Autodesk Inventor part; units mm, degrees
(part 2 of 2)
  line L952 (0.1814, -11.5919) -> (0.1714, -11.711)
  line L953 (0.1714, -11.711) -> (0.1647, -11.8346)
  line L954 (0.1647, -11.8346) -> (0.1634, -11.9625)
  line L955 (-2.9506, -10.7687) -> (-2.9407, -10.8745)
  line L956 (-2.9924, -10.5673) -> (-2.9697, -10.6658)
  line L957 (0.5555, -10.738) -> (0.49, -10.8119)
  line L958 (0.49, -10.8119) -> (0.4304, -10.8914)
  line L959 (0.4304, -10.8914) -> (0.3766, -10.9764)
  line L960 (0.3766, -10.9764) -> (0.331, -11.0665)
  line L961 (0.331, -11.0665) -> (0.2878, -11.1619)
  line L962 (0.2878, -11.1619) -> (0.2528, -11.2622)
  line L963 (1.245, -10.4259) -> (1.2243, -10.4284)
  line L964 (1.2656, -10.4234) -> (1.245, -10.4259)
  line L965 (1.2037, -10.4308) -> (1.183, -10.4331)
  line L966 (1.2243, -10.4284) -> (1.2037, -10.4308)
  line L967 (1.183, -10.4331) -> (1.1624, -10.4355)
  line L968 (0.6288, -10.67) -> (0.5555, -10.738)
  line L969 (0.7079, -10.6083) -> (0.6288, -10.67)
  line L970 (0.7968, -10.5532) -> (0.7079, -10.6083)
  line L971 (0.8944, -10.5055) -> (0.7968, -10.5532)
  line L972 (1.0105, -10.4657) -> (0.8944, -10.5055)
  line L973 (1.1624, -10.4355) -> (1.0105, -10.4657)
  line L974 (-3.7234, -9.8177) -> (-3.7039, -9.825)
  line L975 (-3.626, -9.8541) -> (-3.4858, -9.9197)
  line L976 (-3.4858, -9.9197) -> (-3.3825, -9.9862)
  line L977 (-3.3825, -9.9862) -> (-3.2992, -10.0559)
  line L978 (-3.2992, -10.0559) -> (-3.2261, -10.1307)
  line L979 (-3.2261, -10.1307) -> (-3.164, -10.2095)
  line L980 (-3.164, -10.2095) -> (-3.1091, -10.293)
  line L981 (-3.1091, -10.293) -> (-3.0632, -10.3804)
  line L982 (-3.0632, -10.3804) -> (-3.0244, -10.4719)
  line L983 (-3.0244, -10.4719) -> (-2.9924, -10.5673)
  line L984 (-2.9697, -10.6658) -> (-2.9506, -10.7687)
  line L985 (-3.6455, -9.8469) -> (-3.626, -9.8541)
  line L986 (-3.665, -9.8396) -> (-3.6455, -9.8469)
  line L987 (-3.7039, -9.825) -> (-3.6844, -9.8323)
  line L988 (-3.6844, -9.8323) -> (-3.665, -9.8396)
  line L989 (-2.9407, -10.8745) -> (-2.9384, -10.9833)
  line L990 (-2.7491, -14.0774) -> (-2.693, -14.2225)
  line L991 (-2.6334, -14.3678) -> (-2.5704, -14.5132)
  line L992 (-2.5704, -14.5132) -> (-2.504, -14.6587)
  line L993 (-2.504, -14.6587) -> (-2.3621, -14.6822)
  line L994 (-2.3621, -14.6822) -> (-2.22, -14.7044)
  line L995 (-2.22, -14.7044) -> (-2.0777, -14.7251)
  line L996 (-2.0777, -14.7251) -> (-1.9352, -14.7446)
  line L997 (-1.9352, -14.7446) -> (-1.7925, -14.7626)
  line L998 (-1.0768, -14.832) -> (-1.2202, -14.8209)
  line L999 (-1.2202, -14.8209) -> (-1.3635, -14.8084)
  line L1000 (-1.3635, -14.8084) -> (-1.5066, -14.7945)
  line L1001 (-1.5066, -14.7945) -> (-1.6496, -14.7792)
  line L1002 (-1.6496, -14.7792) -> (-1.7925, -14.7626)
  line L1003 (-2.8017, -13.9324) -> (-2.7491, -14.0774)
  line L1004 (3.5714, -13.2094) -> (3.6719, -13.3187)
  line L1005 (6.0773, -12.5539) -> (6.0676, -12.7049)
  line L1006 (6.0546, -12.8571) -> (6.0381, -13.0104)
  line L1007 (6.0381, -13.0104) -> (6.0184, -13.1648)
  line L1008 (6.0184, -13.1648) -> (5.9953, -13.3201)
  line L1009 (6.0676, -12.7049) -> (6.0546, -12.8571)
  line L1010 (5.9953, -13.3201) -> (5.9689, -13.4764)
  line L1011 (5.9689, -13.4764) -> (5.9393, -13.6335)
  line L1012 (6.0835, -12.4041) -> (6.0773, -12.5539)
  line L1013 (6.0862, -12.2556) -> (6.0835, -12.4041)
  line L1014 (6.0854, -12.1085) -> (6.0862, -12.2556)
  line L1015 (6, -11.2615) -> (6.0246, -11.3978)
  line L1016 (6.0246, -11.3978) -> (6.0447, -11.5363)
  line L1017 (6.0447, -11.5363) -> (6.0607, -11.6767)
  line L1018 (6.0607, -11.6767) -> (6.0727, -11.819)
  line L1019 (6.0727, -11.819) -> (6.0809, -11.963)
  line L1020 (6.0809, -11.963) -> (6.0854, -12.1085)
  line L1021 (2.6723, -11.5301) -> (2.7042, -11.654)
  line L1022 (2.7042, -11.654) -> (2.7296, -11.7839)
  line L1023 (2.7296, -11.7839) -> (2.7506, -11.9191)
  line L1024 (2.7506, -11.9191) -> (2.7948, -12.0443)
  line L1025 (2.7948, -12.0443) -> (2.8489, -12.1672)
  line L1026 (2.8489, -12.1672) -> (2.9098, -12.2884)
  line L1027 (2.9098, -12.2884) -> (2.9767, -12.4081)
  line L1028 (2.9767, -12.4081) -> (3.0487, -12.5264)
  line L1029 (3.0487, -12.5264) -> (3.1254, -12.6434)
  line L1030 (3.1254, -12.6434) -> (3.2066, -12.7592)
  line L1031 (3.2066, -12.7592) -> (3.2919, -12.8736)
  line L1032 (2.598, -11.2985) -> (2.6362, -11.4117)
  line L1033 (2.6362, -11.4117) -> (2.6723, -11.5301)
  line L1034 (2.5533, -11.1915) -> (2.598, -11.2985)
  line L1035 (5.704, -10.5164) -> (5.7711, -10.6304)
  line L1036 (5.7711, -10.6304) -> (5.845, -10.7456)
  line L1037 (5.845, -10.7456) -> (5.8949, -10.8686)
  line L1038 (5.8949, -10.8686) -> (5.9359, -10.9964)
  line L1039 (5.9359, -10.9964) -> (5.9707, -11.1276)
  line L1040 (5.9707, -11.1276) -> (6, -11.2615)
  line L1041 (3.2919, -12.8736) -> (3.3813, -12.9868)
  line L1042 (3.3813, -12.9868) -> (3.4745, -13.0987)
  line L1043 (3.4745, -13.0987) -> (3.5714, -13.2094)
  line L1044 (3.6719, -13.3187) -> (3.7758, -13.4267)
  line L1045 (3.7758, -13.4267) -> (3.8832, -13.5333)
  line L1046 (3.8832, -13.5333) -> (3.9939, -13.6386)
  line L1047 (4.225, -13.8449) -> (4.3453, -13.9459)
  line L1048 (2.5024, -11.0908) -> (2.5533, -11.1915)
  line L1049 (5.4577, -9.8547) -> (5.4815, -9.961)
  line L1050 (5.4815, -9.961) -> (5.5101, -10.0701)
  line L1051 (5.5101, -10.0701) -> (5.5476, -10.1798)
  line L1052 (5.5476, -10.1798) -> (5.5941, -10.2899)
  line L1053 (5.5941, -10.2899) -> (5.6456, -10.4025)
  line L1054 (5.6456, -10.4025) -> (5.704, -10.5164)
  line L1055 (2.3918, -10.9064) -> (2.4497, -10.9955)
  line L1056 (2.2612, -10.7475) -> (2.3271, -10.8242)
  line L1057 (5.4821, -9.2499) -> (5.4584, -9.3457)
  line L1058 (5.4584, -9.3457) -> (5.4426, -9.4438)
  line L1059 (5.4426, -9.4438) -> (5.4344, -9.5441)
  line L1060 (5.4344, -9.5441) -> (5.4359, -9.6451)
  line L1061 (5.4359, -9.6451) -> (5.442, -9.7497)
  line L1062 (5.442, -9.7497) -> (5.4577, -9.8547)
  line L1063 (5.9476, -8.6531) -> (5.9304, -8.6649)
  line L1064 (5.9647, -8.6413) -> (5.9476, -8.6531)
  line L1065 (5.9132, -8.6766) -> (5.896, -8.6883)
  line L1066 (5.9304, -8.6649) -> (5.9132, -8.6766)
  line L1067 (5.896, -8.6883) -> (5.8788, -8.7)
  line L1068 (5.5154, -9.1556) -> (5.4821, -9.2499)
  line L1069 (5.5568, -9.0642) -> (5.5154, -9.1556)
  line L1070 (5.6099, -8.9741) -> (5.5568, -9.0642)
  line L1071 (5.6741, -8.8865) -> (5.6099, -8.9741)
  line L1072 (5.7584, -8.7973) -> (5.6741, -8.8865)
  line L1073 (5.8788, -8.7) -> (5.7584, -8.7973)
  line L1074 (1.2656, -10.4234) -> (1.2863, -10.4209)
  line L1075 (1.3688, -10.4104) -> (1.5234, -10.4034)
  line L1076 (1.5234, -10.4034) -> (1.6458, -10.4143)
  line L1077 (1.6458, -10.4143) -> (1.7519, -10.4373)
  line L1078 (1.7519, -10.4373) -> (1.8514, -10.4695)
  line L1079 (1.8514, -10.4695) -> (1.943, -10.5104)
  line L1080 (1.943, -10.5104) -> (2.0304, -10.5589)
  line L1081 (2.0304, -10.5589) -> (2.1117, -10.615)
  line L1082 (2.1117, -10.615) -> (2.1885, -10.6779)
  line L1083 (2.1885, -10.6779) -> (2.2612, -10.7475)
  line L1084 (2.3271, -10.8242) -> (2.3918, -10.9064)
  line L1085 (1.3482, -10.4131) -> (1.3688, -10.4104)
  line L1086 (1.3275, -10.4157) -> (1.3482, -10.4131)
  line L1087 (1.2863, -10.4209) -> (1.3069, -10.4183)
  line L1088 (1.3069, -10.4183) -> (1.3275, -10.4157)
  line L1089 (2.4497, -10.9955) -> (2.5024, -11.0908)
  line L1090 (4.1079, -13.7425) -> (4.225, -13.8449)
  line L1091 (4.3453, -13.9459) -> (4.4687, -14.0453)
  line L1092 (4.4687, -14.0453) -> (4.595, -14.1433)
  line L1093 (4.595, -14.1433) -> (4.7316, -14.0982)
  line L1094 (4.7316, -14.0982) -> (4.8677, -14.0518)
  line L1095 (4.8677, -14.0518) -> (5.0034, -14.004)
  line L1096 (5.0034, -14.004) -> (5.1386, -13.955)
  line L1097 (5.1386, -13.955) -> (5.2733, -13.9046)
  line L1098 (5.9393, -13.6335) -> (5.8072, -13.6903)
  line L1099 (5.8072, -13.6903) -> (5.6745, -13.7458)
  line L1100 (5.6745, -13.7458) -> (5.5413, -13.8)
  line L1101 (5.5413, -13.8) -> (5.4076, -13.853)
  line L1102 (5.4076, -13.853) -> (5.2733, -13.9046)
  line L1103 (3.9939, -13.6386) -> (4.1079, -13.7425)
  line L1104 (9.301, -10.0366) -> (9.4408, -10.0867)
  line L1105 (11.2152, -8.2916) -> (11.2769, -8.4299)
  line L1106 (11.336, -8.5707) -> (11.3927, -8.7141)
  line L1107 (11.3927, -8.7141) -> (11.447, -8.8599)
  line L1108 (11.447, -8.8599) -> (11.4987, -9.0082)
  line L1109 (11.2769, -8.4299) -> (11.336, -8.5707)
  line L1110 (11.4987, -9.0082) -> (11.548, -9.1588)
  line L1111 (11.548, -9.1588) -> (11.5948, -9.3117)
  line L1112 (11.1511, -8.1561) -> (11.2152, -8.2916)
  line L1113 (11.0845, -8.0234) -> (11.1511, -8.1561)
  line L1114 (11.0155, -7.8936) -> (11.0845, -8.0234)
  line L1115 (10.5462, -7.1832) -> (10.6313, -7.2925)
  line L1116 (10.6313, -7.2925) -> (10.7135, -7.4057)
  line L1117 (10.7135, -7.4057) -> (10.793, -7.5227)
  line L1118 (10.793, -7.5227) -> (10.8697, -7.6431)
  line L1119 (10.8697, -7.6431) -> (10.9439, -7.7667)
  line L1120 (10.9439, -7.7667) -> (11.0155, -7.8936)
  line L1121 (7.7245, -8.9675) -> (7.8103, -9.0624)
  line L1122 (7.8103, -9.0624) -> (7.8932, -9.1656)
  line L1123 (7.8932, -9.1656) -> (7.9747, -9.2756)
  line L1124 (7.9747, -9.2756) -> (8.072, -9.3659)
  line L1125 (8.072, -9.3659) -> (8.1769, -9.4496)
  line L1126 (8.1769, -9.4496) -> (8.2872, -9.5285)
  line L1127 (8.2872, -9.5285) -> (8.402, -9.6035)
  line L1128 (8.402, -9.6035) -> (8.5208, -9.6748)
  line L1129 (8.5208, -9.6748) -> (8.6431, -9.7428)
  line L1130 (8.6431, -9.7428) -> (8.7688, -9.8075)
  line L1131 (8.7688, -9.8075) -> (8.8975, -9.8692)
  line L1132 (7.5511, -8.7969) -> (7.6376, -8.8795)
  line L1133 (7.6376, -8.8795) -> (7.7245, -8.9675)
  line L1134 (7.4618, -8.723) -> (7.5511, -8.7969)
  line L1135 (9.9378, -6.661) -> (10.0502, -6.7308)
  line L1136 (10.0502, -6.7308) -> (10.1692, -6.7985)
  line L1137 (10.1692, -6.7985) -> (10.2706, -6.8842)
  line L1138 (10.2706, -6.8842) -> (10.3663, -6.9783)
  line L1139 (10.3663, -6.9783) -> (10.458, -7.0783)
  line L1140 (10.458, -7.0783) -> (10.5462, -7.1832)
  line L1141 (8.8975, -9.8692) -> (9.0293, -9.9279)
  line L1142 (9.0293, -9.9279) -> (9.1638, -9.9837)
  line L1143 (9.1638, -9.9837) -> (9.301, -10.0366)
  line L1144 (9.4408, -10.0867) -> (9.583, -10.134)
  line L1145 (9.583, -10.134) -> (9.7277, -10.1785)
  line L1146 (9.7277, -10.1785) -> (9.8746, -10.2203)
  line L1147 (10.1751, -10.2956) -> (10.3285, -10.3291)
  line L1148 (7.3699, -8.6575) -> (7.4618, -8.723)
  line L1149 (9.4122, -6.1896) -> (9.4827, -6.2726)
  line L1150 (9.4827, -6.2726) -> (9.5588, -6.3559)
  line L1151 (9.5588, -6.3559) -> (9.643, -6.4357)
  line L1152 (9.643, -6.4357) -> (9.7353, -6.5116)
  line L1153 (9.7353, -6.5116) -> (9.8332, -6.5873)
  line L1154 (9.8332, -6.5873) -> (9.9378, -6.661)
  line L1155 (7.1863, -8.5456) -> (7.279, -8.5975)
  line L1156 (6.9968, -8.4656) -> (7.0907, -8.5029)
  line L1157 (9.1528, -5.6427) -> (9.1763, -5.7386)
  line L1158 (9.1763, -5.7386) -> (9.208, -5.8328)
  line L1159 (9.208, -5.8328) -> (9.2473, -5.9254)
  line L1160 (9.2473, -5.9254) -> (9.2956, -6.0141)
  line L1161 (9.2956, -6.0141) -> (9.3496, -6.1039)
  line L1162 (9.3496, -6.1039) -> (9.4122, -6.1896)
  line L1163 (9.2876, -4.898) -> (9.2779, -4.9164)
  line L1164 (9.2973, -4.8796) -> (9.2876, -4.898)
  line L1165 (9.2681, -4.9347) -> (9.2583, -4.9531)
  line L1166 (9.2779, -4.9164) -> (9.2681, -4.9347)
  line L1167 (9.2583, -4.9531) -> (9.2485, -4.9714)
  line L1168 (9.1384, -5.5437) -> (9.1528, -5.6427)
  line L1169 (9.1326, -5.4436) -> (9.1384, -5.5437)
  line L1170 (9.1378, -5.3391) -> (9.1326, -5.4436)
  line L1171 (9.1539, -5.2318) -> (9.1378, -5.3391)
  line L1172 (9.1871, -5.1135) -> (9.1539, -5.2318)
  line L1173 (9.2485, -4.9714) -> (9.1871, -5.1135)
  line L1174 (5.9647, -8.6413) -> (5.9818, -8.6295)
  line L1175 (6.0499, -8.5819) -> (6.1836, -8.5038)
  line L1176 (6.1836, -8.5038) -> (6.297, -8.4566)
  line L1177 (6.297, -8.4566) -> (6.4016, -8.4276)
  line L1178 (6.4016, -8.4276) -> (6.5047, -8.4099)
  line L1179 (6.5047, -8.4099) -> (6.6048, -8.4036)
  line L1180 (6.6048, -8.4036) -> (6.7048, -8.4059)
  line L1181 (6.7048, -8.4059) -> (6.8028, -8.4177)
  line L1182 (6.8028, -8.4177) -> (6.9001, -8.4378)
  line L1183 (6.9001, -8.4378) -> (6.9968, -8.4656)
  line L1184 (7.0907, -8.5029) -> (7.1863, -8.5456)
  line L1185 (6.0329, -8.5938) -> (6.0499, -8.5819)
  line L1186 (6.0159, -8.6057) -> (6.0329, -8.5938)
  line L1187 (5.9818, -8.6295) -> (5.9989, -8.6176)
  line L1188 (5.9989, -8.6176) -> (6.0159, -8.6057)
  line L1189 (7.279, -8.5975) -> (7.3699, -8.6575)
  line L1190 (10.0238, -10.2593) -> (10.1751, -10.2956)
  line L1191 (10.3285, -10.3291) -> (10.484, -10.3598)
  line L1192 (10.484, -10.3598) -> (10.6414, -10.3878)
  line L1193 (10.6414, -10.3878) -> (10.7414, -10.2844)
  line L1194 (10.7414, -10.2844) -> (10.8403, -10.1801)
  line L1195 (10.8403, -10.1801) -> (10.9383, -10.0748)
  line L1196 (10.9383, -10.0748) -> (11.0352, -9.9685)
  line L1197 (11.0352, -9.9685) -> (11.1311, -9.8613)
  line L1198 (11.5948, -9.3117) -> (11.5042, -9.4234)
  line L1199 (11.5042, -9.4234) -> (11.4125, -9.5342)
  line L1200 (11.4125, -9.5342) -> (11.3198, -9.6442)
  line L1201 (11.3198, -9.6442) -> (11.226, -9.7532)
  line L1202 (11.226, -9.7532) -> (11.1311, -9.8613)
  line L1203 (9.8746, -10.2203) -> (10.0238, -10.2593)
  line L1204 (12.8999, -4.5646) -> (13.0469, -4.544)
  line L1205 (13.7839, -2.1299) -> (13.9027, -2.2236)
  line L1206 (14.0206, -2.3209) -> (14.1374, -2.4215)
  line L1207 (14.1374, -2.4215) -> (14.2532, -2.5254)
  line L1208 (14.2532, -2.5254) -> (14.3679, -2.6326)
  line L1209 (13.9027, -2.2236) -> (14.0206, -2.3209)
  line L1210 (14.3679, -2.6326) -> (14.4816, -2.7431)
  line L1211 (14.4816, -2.7431) -> (14.594, -2.8567)
  line L1212 (13.6642, -2.0397) -> (13.7839, -2.1299)
  line L1213 (13.5435, -1.9531) -> (13.6642, -2.0397)
  line L1214 (13.422, -1.8703) -> (13.5435, -1.9531)
  line L1215 (12.6764, -1.4593) -> (12.8025, -1.5165)
  line L1216 (12.8025, -1.5165) -> (12.928, -1.5786)
  line L1217 (12.928, -1.5786) -> (13.0526, -1.6452)
  line L1218 (13.0526, -1.6452) -> (13.1766, -1.7162)
  line L1219 (13.1766, -1.7162) -> (13.2997, -1.7913)
  line L1220 (13.2997, -1.7913) -> (13.422, -1.8703)
  line L1221 (11.0071, -4.3506) -> (11.1272, -4.3948)
  line L1222 (11.1272, -4.3948) -> (11.2485, -4.4476)
  line L1223 (11.2485, -4.4476) -> (11.3718, -4.5071)
  line L1224 (11.3718, -4.5071) -> (11.4999, -4.5418)
  line L1225 (11.4999, -4.5418) -> (11.6317, -4.5672)
  line L1226 (11.6317, -4.5672) -> (11.7661, -4.5858)
  line L1227 (11.7661, -4.5858) -> (11.9026, -4.5989)
  line L1228 (11.9026, -4.5989) -> (12.0409, -4.6068)
  line L1229 (12.0409, -4.6068) -> (12.1808, -4.6101)
  line L1230 (12.1808, -4.6101) -> (12.3221, -4.6091)
  line L1231 (12.3221, -4.6091) -> (12.4648, -4.6038)
  line L1232 (10.7743, -4.2801) -> (10.8892, -4.313)
  line L1233 (10.8892, -4.313) -> (11.0071, -4.3506)
  line L1234 (10.6609, -4.2561) -> (10.7743, -4.2801)
  line L1235 (11.895, -1.2797) -> (12.027, -1.2893)
  line L1236 (12.027, -1.2893) -> (12.1638, -1.2939)
  line L1237 (12.1638, -1.2939) -> (12.2934, -1.3227)
  line L1238 (12.2934, -1.3227) -> (12.4219, -1.3615)
  line L1239 (12.4219, -1.3615) -> (12.5495, -1.4074)
  line L1240 (12.5495, -1.4074) -> (12.6764, -1.4593)
  line L1241 (12.4648, -4.6038) -> (12.6087, -4.5946)
  line L1242 (12.6087, -4.5946) -> (12.7538, -4.5815)
  line L1243 (12.7538, -4.5815) -> (12.8999, -4.5646)
  line L1244 (13.0469, -4.544) -> (13.1949, -4.5198)
  line L1245 (13.1949, -4.5198) -> (13.3436, -4.492)
  line L1246 (13.3436, -4.492) -> (13.4932, -4.4607)
  line L1247 (13.7942, -4.3877) -> (13.9456, -4.346)
  line L1248 (10.5491, -4.2408) -> (10.6609, -4.2561)
  line L1249 (11.2106, -1.1065) -> (11.3115, -1.1473)
  line L1250 (11.3115, -1.1473) -> (11.4177, -1.1857)
  line L1251 (11.4177, -1.1857) -> (11.5292, -1.2172)
  line L1252 (11.5292, -1.2172) -> (11.6463, -1.2415)
  line L1253 (11.6463, -1.2415) -> (11.7682, -1.263)
  line L1254 (11.7682, -1.263) -> (11.895, -1.2797)
  line L1255 (10.3345, -4.2271) -> (10.4407, -4.23)
  line L1256 (10.1296, -4.2444) -> (10.23, -4.2337)
  line L1257 (10.7267, -0.7429) -> (10.7921, -0.8168)
  line L1258 (10.7921, -0.8168) -> (10.8639, -0.8855)
  line L1259 (10.8639, -0.8855) -> (10.9417, -0.9492)
  line L1260 (10.9417, -0.9492) -> (11.0257, -1.0054)
  line L1261 (11.0257, -1.0054) -> (11.1152, -1.0597)
  line L1262 (11.1152, -1.0597) -> (11.2106, -1.1065)
  line L1263 (10.5, -0.0208) -> (10.4999, -0.0416)
  line L1264 (10.5, 0) -> (10.5, -0.0208)
  line L1265 (10.4998, -0.0624) -> (10.4997, -0.0832)
  line L1266 (10.4999, -0.0416) -> (10.4998, -0.0624)
  line L1267 (10.4997, -0.0832) -> (10.4995, -0.104)
  line L1268 (10.668, -0.6619) -> (10.7267, -0.7429)
  line L1269 (10.6163, -0.5759) -> (10.668, -0.6619)
  line L1270 (10.5723, -0.481) -> (10.6163, -0.5759)
  line L1271 (10.5367, -0.3785) -> (10.5723, -0.481)
  line L1272 (10.5112, -0.2583) -> (10.5367, -0.3785)
  line L1273 (10.4995, -0.104) -> (10.5112, -0.2583)
  line L1274 (9.2973, -4.8796) -> (9.3069, -4.8612)
  line L1275 (9.3451, -4.7873) -> (9.4272, -4.656)
  line L1276 (9.4272, -4.656) -> (9.5057, -4.5616)
  line L1277 (9.5057, -4.5616) -> (9.5849, -4.4873)
  line L1278 (9.5849, -4.4873) -> (9.6679, -4.4237)
  line L1279 (9.6679, -4.4237) -> (9.7536, -4.3716)
  line L1280 (9.7536, -4.3716) -> (9.8432, -4.3272)
  line L1281 (9.8432, -4.3272) -> (9.9355, -4.2921)
  line L1282 (9.9355, -4.2921) -> (10.031, -4.2646)
  line L1283 (10.031, -4.2646) -> (10.1296, -4.2444)
  line L1284 (10.23, -4.2337) -> (10.3345, -4.2271)
  line L1285 (9.3356, -4.8058) -> (9.3451, -4.7873)
  line L1286 (9.3261, -4.8243) -> (9.3356, -4.8058)
  line L1287 (9.3069, -4.8612) -> (9.3165, -4.8427)
  line L1288 (9.3165, -4.8427) -> (9.3261, -4.8243)
  line L1289 (10.4407, -4.23) -> (10.5491, -4.2408)
  line L1290 (13.6434, -4.4259) -> (13.7942, -4.3877)
  line L1291 (13.9456, -4.346) -> (14.0976, -4.301)
  line L1292 (14.0976, -4.301) -> (14.25, -4.2527)
  line L1293 (14.25, -4.2527) -> (14.2904, -4.1147)
  line L1294 (14.2904, -4.1147) -> (14.3296, -3.9762)
  line L1295 (14.3296, -3.9762) -> (14.3673, -3.8375)
  line L1296 (14.3673, -3.8375) -> (14.4038, -3.6983)
  line L1297 (14.4038, -3.6983) -> (14.4389, -3.5589)
  line L1298 (14.594, -2.8567) -> (14.5657, -2.9978)
  line L1299 (14.5657, -2.9978) -> (14.536, -3.1385)
  line L1300 (14.536, -3.1385) -> (14.505, -3.2789)
  line L1301 (14.505, -3.2789) -> (14.4726, -3.4191)
  line L1302 (14.4726, -3.4191) -> (14.4389, -3.5589)
  line L1303 (13.4932, -4.4607) -> (13.6434, -4.4259)
  point P0 (13.8131, 7.2497)
  point P1 (8.8618, 12.8385)
  point P2 (1.8804, 15.4863)
  point P3 (-5.5318, 14.5863)
  point P4 (-11.6768, 10.3447)
  point P5 (-15.1467, 3.7333)
  point P6 (-15.1467, -3.7333)
  point P7 (-11.6768, -10.3447)
  point P8 (-5.5318, -14.5863)
  point P9 (1.8804, -15.4863)
  point P10 (8.8618, -12.8385)
  point P11 (13.8131, -7.2497)
  point P12 (1.2243, -10.4284)
  point P13 (1.245, -10.4259)
  point P14 (1.3069, -10.4183)
  point P15 (5.9304, -8.6649)
  point P16 (5.9476, -8.6531)
  point P17 (5.9989, -8.6176)
  point P18 (9.2779, -4.9164)
  point P19 (9.2876, -4.898)
  point P20 (9.3165, -4.8427)
  point P21 (10.4999, -0.0416)
  point P22 (10.4999, 0.0416)
  point P23 (9.3165, 4.8427)
  point P24 (9.3069, 4.8612)
  point P25 (9.2779, 4.9164)
  point P26 (5.9989, 8.6176)
  point P27 (5.9818, 8.6295)
  point P28 (5.9304, 8.6649)
  point P29 (1.3069, 10.4183)
  point P30 (1.2863, 10.4209)
  point P31 (1.2243, 10.4284)
  point P32 (-3.6844, 9.8323)
  point P33 (-3.7039, 9.825)
  point P34 (-3.7622, 9.8028)
  point P35 (-7.8317, 6.9939)
  point P36 (-7.8456, 6.9783)
  point P37 (-7.8869, 6.9316)
  point P38 (-10.1849, 2.5532)
  point P39 (-10.1899, 2.533)
  point P40 (-10.2048, 2.4724)
  point P41 (0, -12.999)
  point P42 (-10.2048, -2.4724)
  point P43 (-10.1998, -2.4926)
  point P44 (-10.1849, -2.5532)
  point P45 (-7.8869, -6.9316)
  point P46 (-7.8731, -6.9472)
  point P47 (-7.8317, -6.9939)
  point P48 (-3.7622, -9.8028)
  point P49 (-3.7428, -9.8103)
  point P50 (-3.6844, -9.8323)
  dimension "d26" = 360
  constraints: 2608 end point, 99 symmetric about line, 1 centre point, 1 point on line, 3901 other
extrude "押し出し5" add sketch "スケッチ5" against normal blind 3 contours L697 L696 L695 L694 L693 L692 L691 L647 L690 L703 L646 L645 L644 L604 L643 L642 L641 L631 L630 L629 L628 L627 L626 L625 L624 L623 L622 L621 L633 L632 L634 L648 L689 L655 L684 L656 L683 L682 L681 L680 L679 L678 L677 L676 L675 L685 L686 L688 L687 L674 L564 L563 L566 L565 L567 L573 L572 L571 L570 L569 L568 L557 L558 L559 L560 L561 L562 L549 L550 L551 L552 L553 L554 L535 L536 L537 L538 L539 L540 L515 L516 L517 L518 L519 L520 L514 L513 L512 L505 L509 L506 L507 L508 L510 L511 L598 L599 L600 L601 L602 L597 L596 L595 L594 L593 L592 L591 L547 L590 L603 L546 L545 L544 L504 L543 L542 L541 L531 L530 L529 L528 L527 L526 L525 L524 L523 L522 L521 L533 L532 L534 L548 L589 L555 L584 L556 L583 L582 L581 L580 L579 L578 L577 L576 L575 L585 L586 L588 L587 L574 L464 L463 L466 L465 L467 L473 L472 L471 L470 L469 L468 L457 L458 L459 L460 L461 L462 L449 L450 L451 L452 L453 L454 L435 L436 L437 L438 L439 L440 L415 L416 L417 L418 L419 L420 L414 L413 L412 L405 L409 L406 L407 L408 L410 L411 L498 L499 L500 L501 L502 L497 L496 L495 L494 L493 L492 L491 L447 L490 L503 L446 L445 L444 L404 L443 L442 L441 L431 L430 L429 L428 L427 L426 L425 L424 L423 L422 L421 L433 L432 L434 L448 L489 L455 L484 L456 L483 L482 L481 L480 L479 L478 L477 L476 L475 L485 L486 L488 L487 L474 L364 L363 L366 L365 L367 L373 L372 L371 L370 L369 L368 L357 L358 L359 L360 L361 L362 L349 L350 L351 L352 L353 L354 L335 L336 L337 L338 L339 L340 L315 L316 L317 L318 L319 L320 L314 L313 L312 L305 L309 L306 L307 L308 L310 L311 L398 L399 L400 L401 L402 L397 L396 L395 L394 L393 L392 L391 L347 L390 L403 L346 L345 L344 L304 L343 L342 L341 L331 L330 L329 L1 L0 | L1 L329 L328 L327 L326 L325 L324 L323 L322 L321 L333 L332 L334 L348 L389 L355 L384 L356 L383 L382 L381 L380 L379 L378 L377 L376 L375 L385 L386 L388 L387 L374 L264 L263 L266 L265 L267 L273 L272 L271 L270 L269 L268 L257 L258 L259 L260 L261 L262 L249 L250 L251 L252 L253 L254 L235 L236 L237 L238 L239 L240 L215 L216 L217 L218 L219 L220 L214 L213 L212 L205 L209 L206 L207 L208 L210 L211 L298 L299 L300 L301 L302 L297 L296 L295 L294 L293 L292 L291 L247 L290 L303 L246 L245 L244 L204 L243 L242 L241 L231 L230 L229 L228 L227 L226 L225 L224 L223 L222 L221 L233 L232 L234 L248 L289 L255 L284 L256 L283 L282 L281 L280 L279 L278 L277 L276 L275 L285 L286 L288 L287 L274 L164 L163 L166 L165 L167 L173 L172 L171 L170 L169 L168 L157 L158 L159 L160 L161 L162 L149 L150 L151 L152 L153 L154 L135 L136 L137 L138 L139 L140 L115 L116 L117 L118 L119 L120 L114 L113 L112 L105 L109 L106 L107 L108 L110 L111 L198 L199 L200 L201 L202 L197 L196 L195 L194 L193 L192 L191 L147 L190 L203 L146 L145 L144 L104 L143 L142 L141 L131 L130 L129 L128 L127 L126 L125 L124 L123 L122 L121 L133 L132 L134 L148 L189 L155 L184 L156 L183 L182 L181 L180 L179 L178 L177 L176 L175 L185 L186 L188 L187 L174 L54 L55 L56 L57 L58 L59 L60 L61 L62 L63 L64 L65 L66 L67 L68 L69 L70 L71 L72 L73 L74 L75 L76 L77 L78 L79 L80 L81 L82 L83 L84 L85 L86 L87 L88 L89 L90 L91 L92 L93 L94 L95 L96 L97 L98 L99 L100 L101 L102 L103 L51 L50 L49 L48 L47 L46 L45 L44 L43 L42 L41 L40 L39 L38 L37 L36 L35 L34 L33 L32 L31 L30 L29 L28 L27 L26 L25 L24 L23 L22 L21 L20 L19 L18 L17 L16 L15 L14 L13 L12 L11 L10 L9 L8 L7 L6 L5 L4 L3 L2 L0 | L0 L1264 L1263 L1266 L1265 L1267 L1273 L1272 L1271 L1270 L1269 L1268 L1257 L1258 L1259 L1260 L1261 L1262 L1249 L1250 L1251 L1252 L1253 L1254 L1235 L1236 L1237 L1238 L1239 L1240 L1215 L1216 L1217 L1218 L1219 L1220 L1214 L1213 L1212 L1205 L1209 L1206 L1207 L1208 L1210 L1211 L1298 L1299 L1300 L1301 L1302 L1297 L1296 L1295 L1294 L1293 L1292 L1291 L1247 L1290 L1303 L1246 L1245 L1244 L1204 L1243 L1242 L1241 L1231 L1230 L1229 L1228 L1227 L1226 L1225 L1224 L1223 L1222 L1221 L1233 L1232 L1234 L1248 L1289 L1255 L1284 L1256 L1283 L1282 L1281 L1280 L1279 L1278 L1277 L1276 L1275 L1285 L1286 L1288 L1287 L1274 L1164 L1163 L1166 L1165 L1167 L1173 L1172 L1171 L1170 L1169 L1168 L1157 L1158 L1159 L1160 L1161 L1162 L1149 L1150 L1151 L1152 L1153 L1154 L1135 L1136 L1137 L1138 L1139 L1140 L1115 L1116 L1117 L1118 L1119 L1120 L1114 L1113 L1112 L1105 L1109 L1106 L1107 L1108 L1110 L1111 L1198 L1199 L1200 L1201 L1202 L1197 L1196 L1195 L1194 L1193 L1192 L1191 L1147 L1190 L1203 L1146 L1145 L1144 L1104 L1143 L1142 L1141 L1131 L1130 L1129 L1128 L1127 L1126 L1125 L1124 L1123 L1122 L1121 L1133 L1132 L1134 L1148 L1189 L1155 L1184 L1156 L1183 L1182 L1181 L1180 L1179 L1178 L1177 L1176 L1175 L1185 L1186 L1188 L1187 L1174 L1064 L1063 L1066 L1065 L1067 L1073 L1072 L1071 L1070 L1069 L1068 L1057 L1058 L1059 L1060 L1061 L1062 L1049 L1050 L1051 L1052 L1053 L1054 L1035 L1036 L1037 L1038 L1039 L1040 L1015 L1016 L1017 L1018 L1019 L1020 L1014 L1013 L1012 L1005 L1009 L1006 L1007 L1008 L1010 L1011 L1098 L1099 L1100 L1101 L1102 L1097 L1096 L1095 L1094 L1093 L1092 L1091 L1047 L1090 L1103 L1046 L1045 L1044 L1004 L1043 L1042 L1041 L1031 L1030 L1029 L1028 L1027 L1026 L1025 L1024 L1023 L1022 L1021 L1033 L1032 L1034 L1048 L1089 L1055 L1084 L1056 L1083 L1082 L1081 L1080 L1079 L1078 L1077 L1076 L1075 L1085 L1086 L1088 L1087 L1074 L964 L963 L966 L965 L967 L973 L972 L971 L970 L969 L968 L957 L958 L959 L960 L961 L962 L949 L950 L951 L952 L953 L954 L935 L936 L937 L938 L939 L940 L915 L916 L1
extrude "押し出し6" add sketch "スケッチ5" against normal blind 3 contours L0 L1 L916 L917 L918 L919 L920 L914 L913 L912 L905 L909 L906 L907 L908 L910 L911 L998 L999 L1000 L1001 L1002 L997 L996 L995 L994 L993 L992 L991 L947 L990 L1003 L946 L945 L944 L904 L943 L942 L941 L931 L930 L929 L928 L927 L926 L925 L924 L923 L922 L921 L933 L932 L934 L948 L989 L955 L984 L956 L983 L982 L981 L980 L979 L978 L977 L976 L975 L985 L986 L988 L987 L974 L864 L863 L866 L865 L867 L873 L872 L871 L870 L869 L868 L857 L858 L859 L860 L861 L862 L849 L850 L851 L852 L853 L854 L835 L836 L837 L838 L839 L840 L815 L816 L817 L818 L819 L820 L814 L813 L812 L805 L809 L806 L807 L808 L810 L811 L898 L899 L900 L901 L902 L897 L896 L895 L894 L893 L892 L891 L847 L890 L903 L846 L845 L844 L804 L843 L842 L841 L831 L830 L829 L828 L827 L826 L825 L824 L823 L822 L821 L833 L832 L834 L848 L889 L855 L884 L856 L883 L882 L881 L880 L879 L878 L877 L876 L875 L885 L886 L888 L887 L874 L764 L763 L766 L765 L767 L773 L772 L771 L770 L769 L768 L757 L758 L759 L760 L761 L762 L749 L750 L751 L752 L753 L754 L735 L736 L737 L738 L739 L740 L715 L716 L717 L718 L719 L720 L714 L713 L712 L705 L709 L706 L707 L708 L710 L711 L798 L799 L800 L801 L802 L797 L796 L795 L794 L793 L792 L791 L747 L790 L803 L746 L745 L744 L704 L743 L742 L741 L731 L730 L729 L728 L727 L726 L725 L724 L723 L722 L721 L733 L732 L734 L748 L789 L755 L784 L756 L783 L782 L781 L780 L779 L778 L777 L776 L775 L785 L786 L788 L787 L774 L664 L663 L666 L665 L667 L673 L672 L671 L670 L669 L668 L657 L658 L659 L660 L661 L662 L649 L650 L651 L652 L653 L654 L635 L636 L637 L638 L639 L640 L615 L616 L617 L618 L619 L620 L614 L613 L612 L605 L609 L606 L607 L608 L610 L611 L698 L699 L700 L701 L702
sketch "スケッチ4" plane through (0, 3, 0) normal (0, 1, 0) x (1, 0, 0)
  circle A0 centre (0, 0) radius 1.75
  dimension "d21" = 3.5
  constraints: 1 centre point, 1 coincident
  measures "d21" diameter of A0
extrude "押し出し4" cut sketch "スケッチ4" against normal through all
sketch "スケッチ6" plane through (0, 3, 0) normal (0, 1, 0) x (1, 0, 0)
  circle A0 centre (5, 0) radius 0.8 projected
  circle A1 centre (-5, 0) radius 0.8 projected
  circle A2 centre (3.5355, 3.5355) radius 0.8 projected
  circle A3 centre (-3.5355, -3.5355) radius 0.8 projected
  circle A4 centre (3.5355, -3.5355) radius 0.8 projected
  circle A5 centre (-3.5355, 3.5355) radius 0.8 projected
  circle A6 centre (0, -5) radius 0.8 projected
  circle A7 centre (0, 5) radius 0.8 projected
  circle A8 centre (0, 0) radius 1.6 projected
  arc A9 (-0.4294, -14.6804) -> (0.4294, -14.6804) centre (0, 0) ccw projected
  arc A10 (-5.5788, -13.5859) -> (-0.4294, -14.6804) centre (0, 0) ccw projected
  arc A11 (-6.3633, -13.2366) -> (-5.5788, -13.5859) centre (0, 0) ccw projected
  arc A12 (-10.6224, -10.1422) -> (-6.3633, -13.2366) centre (0, 0) ccw projected
  arc A13 (-11.197, -9.5041) -> (-10.6224, -10.1422) centre (0, 0) ccw projected
  arc A14 (-13.8293, -4.9448) -> (-11.197, -9.5041) centre (0, 0) ccw projected
  arc A15 (-14.0946, -4.1282) -> (-13.8293, -4.9448) centre (0, 0) ccw projected
  arc A16 (-14.6449, 1.1075) -> (-14.0946, -4.1282) centre (0, 0) ccw projected
  arc A17 (-14.5551, 1.9615) -> (-14.6449, 1.1075) centre (0, 0) ccw projected
  arc A18 (-12.9283, 6.9684) -> (-14.5551, 1.9615) centre (0, 0) ccw projected
  arc A19 (-12.499, 7.7121) -> (-12.9283, 6.9684) centre (0, 0) ccw projected
  arc A20 (-8.9763, 11.6244) -> (-12.499, 7.7121) centre (0, 0) ccw projected
  arc A21 (-8.2816, 12.1291) -> (-8.9763, 11.6244) centre (0, 0) ccw projected
  arc A22 (-3.4722, 14.2704) -> (-8.2816, 12.1291) centre (0, 0) ccw projected
  arc A23 (-2.6323, 14.4489) -> (-3.4722, 14.2704) centre (0, 0) ccw projected
  arc A24 (2.6323, 14.4489) -> (-2.6323, 14.4489) centre (0, 0) ccw projected
  arc A25 (3.4722, 14.2704) -> (2.6323, 14.4489) centre (0, 0) ccw projected
  arc A26 (8.2816, 12.1291) -> (3.4722, 14.2704) centre (0, 0) ccw projected
  arc A27 (8.9763, 11.6244) -> (8.2816, 12.1291) centre (0, 0) ccw projected
  arc A28 (12.499, 7.7121) -> (8.9763, 11.6244) centre (0, 0) ccw projected
  arc A29 (12.9283, 6.9684) -> (12.499, 7.7121) centre (0, 0) ccw projected
  arc A30 (14.5551, 1.9615) -> (12.9283, 6.9684) centre (0, 0) ccw projected
  arc A31 (14.6449, 1.1075) -> (14.5551, 1.9615) centre (0, 0) ccw projected
  arc A32 (14.0946, -4.1282) -> (14.6449, 1.1075) centre (0, 0) ccw projected
  arc A33 (13.8293, -4.9448) -> (14.0946, -4.1282) centre (0, 0) ccw projected
  arc A34 (11.197, -9.5041) -> (13.8293, -4.9448) centre (0, 0) ccw projected
  arc A35 (10.6224, -10.1422) -> (11.197, -9.5041) centre (0, 0) ccw projected
  arc A36 (6.3633, -13.2366) -> (10.6224, -10.1422) centre (0, 0) ccw projected
  arc A37 (5.5788, -13.5859) -> (6.3633, -13.2366) centre (0, 0) ccw projected
  arc A38 (0.4294, -14.6804) -> (5.5788, -13.5859) centre (0, 0) ccw projected
  circle A39 centre (-5, 0) radius 1.1
  circle A40 centre (-3.5355, -3.5355) radius 1.1
  circle A41 centre (0, -5) radius 1.1
  circle A42 centre (3.5355, -3.5355) radius 1.1
  circle A43 centre (5, 0) radius 1.1
  circle A44 centre (3.5355, 3.5355) radius 1.1
  circle A45 centre (0, 5) radius 1.1
  circle A46 centre (-3.5355, 3.5355) radius 1.1
  point P0 (0, 0)
  dimension "d32" = 2.2
  dimension "d35" = 360
  constraints: 8 centre point, 1 coincident, 17 other
  measures "d32" diameter of A39
extrude "押し出し7" cut sketch "スケッチ6" against normal blind 10 contours A0 | A1 | A2 | A3 | A4 | A5 | A6 | A7 | A39 | A40 | A41 | A42 | A43 | A44 | A45 | A46
sketch "スケッチ7" plane through (0, 3, 0) normal (0, 1, 0) x (1, 0, 0)
  circle A0 centre (0, 0) radius 7
  circle A1 centre (5, 0) radius 1.1 projected
  circle A2 centre (5, 0) radius 2
  dimension "d39" = 4
  constraints: 2 centre point, 2 coincident, 1 tangent
  measures "d39" diameter of A2
extrude "押し出し8" cut sketch "スケッチ7" against normal blind 1.5 contours A0 | A2
